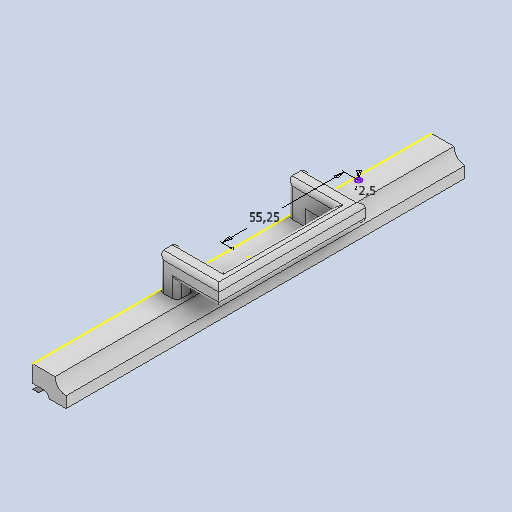
# Autodesk Inventor part: test3
Saved by Autodesk Inventor 2025 (Build 290162000, 162)
## iProperties
Created: 2025-04-20
Part Number: test3
Material: Generic
Document SubType Name: Sheet Metal
Designer: Pravoslav
Density: 1 g/cm^3
Sheet Metal Rule: Default_mm
Appearance: Default
Author: Pravoslav
Autodesk Inventor part; units mm, degrees
ref_plane "YZ Plane" through (0, 0, 0) normal (1, 0, 0) x (0, 1, 0)
ref_plane "XZ Plane" through (0, 0, 0) normal (0, 1, 0) x (-1, 0, 0)
ref_plane "XY Plane" through (0, 0, 0) normal (0, 0, 1) x (1, 0, 0)
sketch "Sketch1" plane through (0, 0, 0) normal (0, 1, 0) x (-1, 0, 0)
  line L0 (7.5, 90) -> (-7.5, 90)
  line L1 (-7.5, 90) -> (-7.5, -90)
  line L2 (-7.5, -90) -> (7.5, -90)
  line L3 (7.5, -90) -> (7.5, 90)
  line L4 (7.5, 90) -> (-7.5, -90) construction
  line L5 (-7.5, 90) -> (7.5, -90) construction
  point P0 (0, 0)
  dimension "d0" = 15
  dimension "d1" = 180
  constraints: 12 end point, 2 midpoint, 2 parallel, 1 horizontal, 1 perpendicular
  measures "d0" distance of L2.end L1.end
  measures "d1" distance of L1.end L0.end
extrude "Extrusion1" add sketch "Sketch1" along normal blind 5
sketch "Sketch2" plane through (0, 5, 0) normal (0, 1, 0) x (1, 0, 0)
  line L0 (7.5, 90) -> (-7.5, 90) projected
  line L1 (-7.5, -90) -> (7.5, -90) projected
  line L2 (-7.5, 90) -> (2.5, 90)
  line L3 (2.5, 90) -> (2.5, -90)
  line L4 (2.5, -90) -> (-7.5, -90)
  line L5 (-7.5, -90) -> (-7.5, 90)
  point P0 (0, 0)
  dimension "d4" = 10
  constraints: 8 end point, 2 parallel, 1 horizontal, 1 perpendicular, 1 point on line
  measures "d4" distance of L3.end L4.end
extrude "Extrusion2" add sketch "Sketch2" along normal blind 5
fillet "Fillet1" radius 5 1 edges at (2.5, 5, 0)
sketch "Sketch3" plane through (7.5, 0, -90) normal (0, 0, -1) x (-1, 0, 0)
  line L0 (15, 0) -> (0, 0) projected
  circle A0 centre (10, 0) radius 2.325
  line L1 (15, 0) -> (15, 10) projected
  point P0 (7.5, 0)
  point P1 (7.675, 0)
  point P2 (12.325, 0)
  dimension "d8" = 4.65
  dimension "d9" = 5
  constraints: 1 centre point, 1 point on line
  measures "d8" diameter of A0
  measures "d9" distance from line of L1 A0.centre
extrude "Extrusion3" cut sketch "Sketch3" against normal through all contours L0 A0 picked at (10.6026, 0.6994)
sketch "Sketch4" plane through (0, 10, 0) normal (0, 1, 0) x (1, 0, 0)
  circle A0 centre (-5.7647, 55.25) radius 1.25
  line L0 (-7.5, 90) -> (-7.5, -90) projected
  point P0 (0, 0)
  point P1 (-7.5, 0)
  dimension "d12" = 2.5
  dimension "d13" = 55.25
  constraints: 1 centre point, 1 midpoint
  measures "d12" diameter of A0
  measures "d13" vertical distance of point (-7.5, 0) A0.centre
sketch "Sketch5" plane through (0, 0, 0) normal (0, -1, 0) x (1, 0, 0)
  circle A0 centre (-5.7647, -55.25) radius 1.25 projected
  circle A1 centre (-5.7647, -55.25) radius 1.6333
  point P0 (0, 0)
  constraints: 1 centre point, 1 coincident
extrude "Extrusion4" cut sketch "Sketch5" against normal blind 2 contours A0 | A1
mirror "Mirror1" about plane through (0, 0, 0) normal (0, 0, 1) of "Extrusion4"
sketch "Sketch6" plane through (-7.5, 0, -90) normal (0, 0, -1) x (-1, 0, 0)
  arc A0 (-2.675, 0) -> (-7.325, 0) centre (-5, 0) ccw projected
  line L0 (0, 0.075) -> (-5, 0.075)
  line L1 (-5, 0.075) -> (-5, 2.325)
  line L2 (-5, 2.325) -> (0, 2.325)
  line L3 (0, 2.325) -> (0, 0.075)
  point P0 (-7.5, 0)
  constraints: 8 end point, 2 parallel, 1 horizontal, 1 perpendicular, 1 point on circle
extrude "Extrusion5" cut sketch "Sketch6" against normal blind 12
mirror "Mirror2" about plane through (0, 0, 0) normal (0, 0, 1) of "Extrusion5"
sketch "Sketch7" plane through (0, 10, 0) normal (0, 1, 0) x (1, 0, 0)
  line L0 (-7.5, 90) -> (-7.5, -90) projected
  line L1 (-7.5, 33) -> (0.5, 33)
  line L2 (0.5, 33) -> (0.5, 25)
  line L3 (0.5, 25) -> (-7.5, 25)
  line L4 (-7.5, 25) -> (-7.5, 33)
  line L5 (-7.5, -25) -> (0.5, -25)
  line L6 (0.5, -25) -> (0.5, -33)
  line L7 (0.5, -33) -> (-7.5, -33)
  line L8 (-7.5, -33) -> (-7.5, -25)
  point P0 (0, 0)
  point P1 (-3.5, -25)
  point P2 (-3.5, 25)
  point P3 (-7.5, 25)
  point P4 (-7.5, -25)
  point P5 (-7.5, -33)
  dimension "d18" = 8
  dimension "d19" = 8
  dimension "d20" = 8
  dimension "d21" = 8
  dimension "d22" = 50
  dimension "d23" = 25
  constraints: 16 end point, 4 parallel, 2 horizontal, 2 midpoint, 2 perpendicular, 2 point on line
  measures "d18" distance of L2.end L3.end
  measures "d19" distance of L1.end L2.end
  measures "d20" distance of L6.end L7.end
  measures "d21" distance of L5.end L6.end
  measures "d22" distance of point (-3.5, -25) point (-3.5, 25)
  measures "d23" vertical distance of point (0, 0) point (-3.5, 25)
extrude "Extrusion6" add sketch "Sketch7" along normal blind 15
sketch "Sketch9" plane through (-7.5, 2.325, -90) normal (-1, 0, 0) x (0, 0, 1)
  line L0 (57, 7.675) -> (57, 22.675) projected
  line L1 (57, 22.675) -> (65, 22.675)
  line L2 (65, 22.675) -> (65, 14.675)
  line L3 (65, 14.675) -> (57, 14.675)
  line L4 (57, 14.675) -> (57, 22.675)
  line L5 (115, 22.675) -> (123, 22.675) projected
  line L6 (123, 7.675) -> (123, 22.675) projected
  line L7 (115, 22.675) -> (123, 22.675)
  line L8 (123, 22.675) -> (123, 14.675)
  line L9 (123, 14.675) -> (115, 14.675)
  line L10 (115, 14.675) -> (115, 22.675)
  point P0 (90, -2.325)
  dimension "d28" = 8
  dimension "d29" = 8
  constraints: 16 end point, 4 parallel, 2 horizontal, 2 perpendicular, 2 point on line
  measures "d28" distance of L2.end L3.end
  measures "d29" distance of L1.end L2.end
extrude "Extrusion8" add sketch "Sketch9" against normal blind 21
sketch "Sketch11" plane through (13.5, 2.325, -90) normal (1, 0, 0) x (0, 0, -1)
  line L0 (-123, 7.675) -> (-123, 22.675) projected
  line L1 (-57, 14.675) -> (-65, 14.675) projected
  line L2 (-123, 22.675) -> (-57, 22.675)
  line L3 (-57, 22.675) -> (-57, 14.675)
  line L4 (-57, 14.675) -> (-123, 14.675)
  line L5 (-123, 14.675) -> (-123, 22.675)
  point P0 (-90, -2.325)
  constraints: 8 end point, 2 parallel, 1 horizontal, 1 perpendicular
extrude "Extrusion10" add sketch "Sketch11" along normal blind 6
fillet "Fillet3" radius 2 18 edges at (13.5, 25, 0) (19.5, 25, 0) (13.5, 17, 0) (7, 17, 25) (3, 25, 25) (0.5, 13.5, 25) (-7.5, 17.5, 25) (-7.5, 17.5, 33) (6, 25, 33) (6, 25, -33) (3, 25, -25) (-7.5, 17.5, -33) (-7.5, 17.5, -25) (10, 17, -33) (0.5, 13.5, -33) (19.5, 17, 0) (10, 17, 33) (0.5, 13.5, 33)
sketch "Sketch10" plane through (13.5, 2.325, -90) normal (1, 0, 0) x (0, 0, 1)
  line L0 (65, -22.675) -> (58, -22.675) projected
  line L1 (123, -14.675) -> (115, -14.675) projected
  line L2 (58, 22.75) -> (122, 22.75)
  line L3 (122, 22.75) -> (122, -14.675)
  line L4 (123, 16.75) -> (58, 16.75)
  line L5 (58, 16.75) -> (58, 22.75)
  point P0 (90, 2.325)
  point P1 (65, 22.75)
  point P2 (115, 16.75)
  constraints: 6 end point, 2 horizontal, 1 parallel, 1 perpendicular, 4 other
sketch "Sketch8" plane through (0, 25, 0) normal (0, 1, 0) x (1, 0, 0)
  line L0 (-7.5, 78) -> (-7.5, -78) projected
  line L1 (0.5, -25) -> (0.5, -33) projected
  line L2 (-7.5, 31.8346) -> (-2.5, 31.8346)
  line L3 (-2.5, 31.8346) -> (-2.5, -33)
  line L4 (0.5, -32) -> (-7.5, -32)
  line L5 (-7.5, -32) -> (-7.5, 31.8346)
  point P0 (0, 0)
  point P1 (-2.5, -25)
  constraints: 4 end point, 3 horizontal, 1 point on line, 1 vertical, 6 other
equation "\"BendRadius\" = Thickness"
equation "\"BendReliefWidth\" = Thickness"
equation "\"BendReliefDepth\" = 0.5 * Thickness"
equation "\"CornerReliefSize\" = 4 * Thickness"
equation "\"MinimumRemnant\" = 2 * Thickness"
equation "\"TransitionRadius\" = BendRadius"
equation "\"JacobiRadiusSize\" = BendRadius"
equation "\"GapSize\" = Thickness"
equation "\"Thickness\" = 0.5"
body "Solid1"
